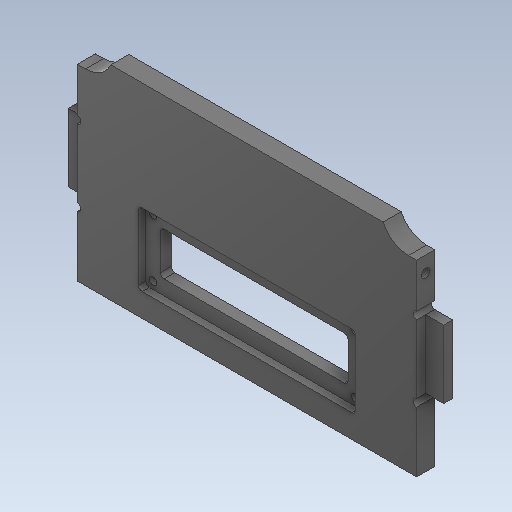
# Autodesk Inventor part: Cockpit_horizontal_frame_05
Saved by Autodesk Inventor 2020.4 (Build 244396000, 396)
## iProperties
Created: 2021-08-14
Part Number: Cockpit_horizontal_frame_05
Material: アセタール樹脂、黒
Document SubType Name: Modeling
Designer: Masato Kubotera
Density: 1.425 g/cm^3
Appearance: 滑らか - 黒
Mass: 37.8231 g
Surface Area: 126.929 cm^2
Volume: 26.5425 cm^3
Description: POM T5
Author: Masato Kubotera
Title: Cockpit_horizontal_frame_05
Autodesk Inventor part; units mm, degrees
ref_plane "YZ Plane" through (0, 0, 0) normal (1, 0, 0) x (0, 1, 0)
ref_plane "XZ Plane" through (0, 0, 0) normal (0, 1, 0) x (-1, 0, 0)
ref_plane "XY Plane" through (0, 0, 0) normal (0, 0, 1) x (1, 0, 0)
sketch "スケッチ1" plane through (0, 0, 0) normal (0, 0, 1) x (1, 0, 0)
  line L0 (-47, 28.25) -> (-37.7144, 28.25)
  line L1 (47, 28.25) -> (47, 23.75)
  line L2 (47, -28.25) -> (-47, -28.25)
  line L3 (-47, -28.25) -> (-47, -11.5167)
  line L4 (-47, 28.25) -> (47, -28.25) construction
  line L5 (47, 28.25) -> (-47, -28.25) construction
  line L6 (0, 28.25) -> (0, -28.25) construction
  line L7 (-52, 9.4167) -> (-52, -9.4167)
  line L8 (-52, 9.4167) -> (-47, 9.4167)
  arc A0 (-47, 9.4167) -> (-47, 11.5167) centre (-47, 10.4667) ccw
  line L9 (-47, 11.5167) -> (-47, 23.75)
  line L10 (-47, -11.5167) -> (-47, 11.5167)
  line L11 (52, 9.4167) -> (52, -9.4167)
  line L12 (52, 9.4167) -> (47, 9.4167)
  arc A1 (47, 11.5167) -> (47, 9.4167) centre (47, 10.4667) ccw
  line L13 (47, 11.5167) -> (47, -11.5167)
  line L14 (47, -11.5167) -> (47, -28.25)
  line L15 (-52, 0) -> (52, 0) construction
  line L16 (-52, -9.4167) -> (-47, -9.4167)
  arc A2 (-47, -11.5167) -> (-47, -9.4167) centre (-47, -10.4667) ccw
  arc A3 (47, -9.4167) -> (47, -11.5167) centre (47, -10.4667) ccw
  line L17 (52, -9.4167) -> (47, -9.4167)
  arc A4 (-47, 24.0838) -> (-37.7144, 28.25) centre (-44.75, 31.5) ccw
  arc A5 (37.7144, 28.25) -> (47, 24.0838) centre (44.75, 31.5) ccw
  line L18 (-47, 24.0838) -> (-47, 28.25)
  line L19 (-37.7144, 28.25) -> (47, 28.25)
  arc A6 (-37.7144, 28.25) -> (-47, 24.0838) centre (-44.75, 31.5) ccw
  arc A7 (47, 24.0838) -> (37.7144, 28.25) centre (44.75, 31.5) ccw
  line L20 (-44.75, 23.75) -> (-47, 23.75)
  line L21 (44.75, 23.75) -> (47, 23.75)
  line L22 (-47, 23.75) -> (-47, 24.0838)
  line L23 (47, 23.75) -> (47, 11.5167)
  line L24 (-30, -1.75) -> (30, -1.75) construction
  line L25 (30, -1.75) -> (30, -21.75) construction
  line L26 (30, -21.75) -> (-30, -21.75) construction
  line L27 (-30, -21.75) -> (-30, -1.75) construction
  line L28 (-30, -1.75) -> (30, -21.75) construction
  line L29 (30, -1.75) -> (-30, -21.75) construction
  circle A8 centre (-28, -3.75) radius 1.05
  line L30 (30, -11.75) -> (-30, -11.75) construction
  circle A9 centre (-28, -19.75) radius 1.05
  circle A10 centre (28, -3.75) radius 1.05
  circle A11 centre (28, -19.75) radius 1.05
  line L31 (-30.05, -1.7) -> (30.05, -1.7)
  line L32 (30.05, -1.7) -> (30.05, -21.8)
  line L33 (30.05, -21.8) -> (-30.05, -21.8)
  line L34 (-30.05, -21.8) -> (-30.05, -1.7)
  line L35 (-30.05, -1.7) -> (30.05, -21.8) construction
  line L36 (30.05, -1.7) -> (-30.05, -21.8) construction
  line L37 (-26, -5.75) -> (26, -5.75)
  line L38 (26, -5.75) -> (26, -17.75)
  line L39 (26, -17.75) -> (-26, -17.75)
  line L40 (-26, -17.75) -> (-26, -5.75)
  line L41 (-26, -5.75) -> (26, -17.75) construction
  line L42 (26, -5.75) -> (-26, -17.75) construction
  point P0 (0, 0)
  point P1 (0, 0)
  point P2 (0, 0)
  point P3 (0, 0)
  point P4 (47, 9.4167)
  point P5 (47, 9.4167)
  point P6 (0, -11.75)
  dimension "d0" = 94
  dimension "d1" = 56.5
  dimension "d10" = 1.05
  dimension "d11" = 5
  dimension "d34" = 18.8333
  dimension "d40" = 31.5
  dimension "d41" = 89.5
  dimension "d42" = 15.5
  dimension "d43" = 52
  dimension "d69" = 60
  dimension "d70" = 20
  dimension "d71" = 2
  dimension "d72" = 2
  dimension "d73" = 2.1
  dimension "d74" = 30
  dimension "d75" = 0.05
  dimension "d76" = 0.05
  dimension "d80" = 4
  dimension "d81" = 4
  constraints: 86 end point, 28 parallel, 18 midpoint, 18 perpendicular, 18 point on circle, 16 symmetric about line, 12 centre point, 9 point on line, 5 horizontal, 1 tangent, 1 vertical, 7 other
  measures "d0" distance of L2.start L2.end
  measures "d1" distance of L2.start L1.start
  measures "d10" radius of A0
  measures "d11" horizontal distance of L7.start L0.start
  measures "d34" distance of L7.start L7.end
  measures "d40" vertical distance of L15.start A4.centre
  measures "d41" distance of A5.centre A4.centre
  measures "d42" diameter of A4
  measures "d43" distance of L2.start L1.end
  measures "d69" distance of L25.end L26.end
  measures "d70" distance of L24.end L25.end
  measures "d71" horizontal distance of A8.centre L24.start
  measures "d72" horizontal distance of L24.start A8.centre
  measures "d73" diameter of A8
  measures "d74" distance between parallel lines of L24 L19
  measures "d75" horizontal distance of L31.start L24.start
  measures "d76" horizontal distance of L24.start L31.start
  measures "d80" horizontal distance of L37.start L24.start
  measures "d81" horizontal distance of L37.start L24.start
extrude "押し出し1" add sketch "スケッチ1" along normal blind 5 contours L19 A5 L21 L23 A1 L13 A3 L14 L2 L3 A2 L10 A0 L9 L20 A4
extrude "押し出し2" add sketch "スケッチ1" along normal blind 2.5 contours L10 L16 L7 L8 | L12 L11 L17 L13
sketch "スケッチ2" plane through (47, 11.5167, 0) normal (1, 0, 0) x (0, 0, -1)
  line L0 (0, -23.0333) -> (-5, -23.0333) projected
  line L1 (-2.5, -23.0333) -> (-2.5, -39.7667)
  line L2 (0, -39.7667) -> (-5, -39.7667) projected
  line L3 (0, -2.1) -> (-2.5, -2.1) projected
  line L4 (0, -20.9333) -> (-2.5, -20.9333) projected
  point P0 (0, -11.5167)
  point P1 (-2.5, 7.9)
  dimension "d67" = 10
  constraints: 2 end point, 2 midpoint, 1 point on line
  measures "d67" distance from line of point (-2.5, 7.9) L3
hole "穴1" at (47, 19.4167, 2.5) direction (-1, 0, 0) diameter 2.459 depth 10 tip angle 118 thread size "M3x0.5" class "6H" standard "ANSI Metric M Profile"
sketch "スケッチ3" plane through (-47, 11.5167, 0) normal (-1, 0, 0) x (0, 0, 1)
  circle A0 centre (2.5, 7.9) radius 1.2295 projected
  circle A1 centre (2.5, -30.9333) radius 1.2295 projected
  point P0 (0, -11.5167)
  point P1 (2.5, 7.9)
  constraints: 1 coincident
hole "穴2" at (-47, 19.4167, 2.5) direction (1, 0, 0) diameter 2.459 depth 10 tip angle 118 thread size "M3x0.5" class "6H" standard "ANSI Metric M Profile"
extrude "押し出し3" add sketch "スケッチ1" along normal blind 3 contours L31 L32 L33 L34
fillet "フィレット1" radius 1 8 edges at (-30.05, -1.7, 4) (-30.05, -21.8, 4) (30.05, -21.8, 4) (30.05, -1.7, 4) (-26, -5.75, 1.5) (-26, -17.75, 1.5) (26, -5.75, 1.5) (26, -17.75, 1.5)
equation "\"d10\" = d4"
equation "\"d4\" = 1.05"
